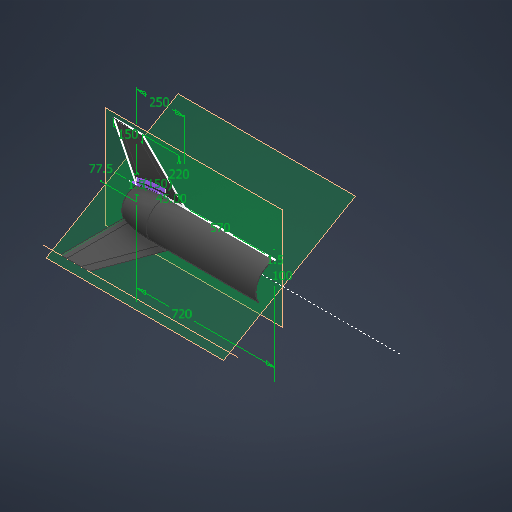
# Autodesk Inventor part: 26P0131-04-0005-AY
Saved by Autodesk Inventor 2026.1 (Build 301233020, 233B)
## iProperties
Created: 2026-01-29
Part Number: 26P0131-04-0005-AY
Material: CFRP
Document SubType Name: Modeling
Designer: User
Density: 1.43 g/cm^3
Appearance: Carbon Fiber
Author: User
Autodesk Inventor part; units mm, degrees
ref_plane "YZ Plane" through (0, 0, 0) normal (1, 0, 0) x (0, 1, 0)
ref_plane "XZ Plane" through (0, 0, 0) normal (0, 1, 0) x (-1, 0, 0)
ref_plane "XY Plane" through (0, 0, 0) normal (0, 0, 1) x (1, 0, 0)
sketch "Sketch3" plane through (0, 0, 0) normal (0, 0, 1) x (1, 0, 0)
  spline S0 degree 4 poles (0, 76) (3.2261, 76.9678) (7.7454, 78.2848) (13.5618, 79.9096) (20.6802, 81.7875) (25.8529, 83.0987) (31.0257, 84.3563) (36.1985, 85.5604) (41.3712, 86.7109) (46.544, 87.808) (51.7168, 88.8516) (56.8895, 89.8416) (62.0623, 90.7781) (67.2351, 91.6611) (72.4079, 92.4906) (77.5807, 93.2666) (82.7535, 93.9891) (87.9263, 94.658) (93.0991, 95.2734) (98.2719, 95.8353) (103.4447, 96.3438) (108.6175, 96.7986) (113.7903, 97.2) (118.9631, 97.5479) (124.1359, 97.8422) (129.3087, 98.083) (136.4207, 98.3405) (142.2404, 98.461) (146.767, 98.5) (150, 98.5) knots 0 0 0 0 0 0.087261 0.122096 0.156887 0.191635 0.226341 0.261008 0.295637 0.33023 0.364788 0.399313 0.433807 0.468271 0.502708 0.537118 0.571504 0.605867 0.64021 0.674533 0.708839 0.74313 0.777407 0.811672 0.845927 0.880174 0.914415 1 1 1 1 1
  spline S1 degree 4 poles (0, 77.5) (3.2261, 78.4678) (7.7454, 79.7848) (13.5618, 81.4096) (20.6802, 83.2875) (25.8529, 84.5987) (31.0257, 85.8563) (36.1985, 87.0604) (41.3712, 88.2109) (46.544, 89.308) (51.7168, 90.3516) (56.8895, 91.3416) (62.0623, 92.2781) (67.2351, 93.1611) (72.4079, 93.9906) (77.5807, 94.7666) (82.7535, 95.4891) (87.9263, 96.158) (93.0991, 96.7734) (98.2719, 97.3353) (103.4447, 97.8438) (108.6175, 98.2986) (113.7903, 98.7) (118.9631, 99.0479) (124.1359, 99.3422) (129.3087, 99.583) (136.4207, 99.8405) (142.2404, 99.961) (146.767, 100) (150, 100) knots 0 0 0 0 0 0.087261 0.122096 0.156887 0.191635 0.226341 0.261008 0.295637 0.33023 0.364788 0.399313 0.433807 0.468271 0.502708 0.537118 0.571504 0.605867 0.64021 0.674533 0.708839 0.74313 0.777407 0.811672 0.845927 0.880174 0.914415 1 1 1 1 1
  line L0 (0, 77.5) -> (0, 76)
  line L1 (150, 100) -> (720, 100)
  line L2 (150, 98.5) -> (720, 98.5)
  line L3 (720, 100) -> (720, 98.5)
  line L4 (0, 0) -> (1383.1618, 0) construction
  line L5 (250, 100) -> (30, 320)
  line L6 (30, 320) -> (-120, 320)
  line L7 (-120, 320) -> (0, 77.5)
  point P0 (5.1724, 77.525)
  point P1 (10.3448, 78.9964)
  point P2 (15.5172, 80.4144)
  point P3 (20.6897, 81.7788)
  point P4 (25.8621, 83.0898)
  point P5 (31.0345, 84.3472)
  point P6 (36.2069, 85.5511)
  point P7 (41.3793, 86.7015)
  point P8 (46.5517, 87.7985)
  point P9 (51.7241, 88.8419)
  point P10 (56.8966, 89.8317)
  point P11 (62.069, 90.7681)
  point P12 (67.2414, 91.651)
  point P13 (72.4138, 92.4804)
  point P14 (77.5862, 93.2562)
  point P15 (82.7586, 93.9786)
  point P16 (87.931, 94.6474)
  point P17 (93.1034, 95.2628)
  point P18 (98.2759, 95.8246)
  point P19 (103.4483, 96.3329)
  point P20 (108.6207, 96.7878)
  point P21 (113.7931, 97.1891)
  point P22 (118.9655, 97.5369)
  point P23 (124.1379, 97.8312)
  point P24 (129.3103, 98.0719)
  point P25 (134.4828, 98.2592)
  point P26 (139.6552, 98.393)
  point P27 (144.8276, 98.4732)
  point P28 (5.1724, 79.025)
  point P29 (10.3448, 80.4964)
  point P30 (15.5172, 81.9144)
  point P31 (20.6897, 83.2788)
  point P32 (25.8621, 84.5898)
  point P33 (31.0345, 85.8472)
  point P34 (36.2069, 87.0511)
  point P35 (41.3793, 88.2015)
  point P36 (46.5517, 89.2985)
  point P37 (51.7241, 90.3419)
  point P38 (56.8966, 91.3317)
  point P39 (62.069, 92.2681)
  point P40 (67.2414, 93.151)
  point P41 (72.4138, 93.9804)
  point P42 (77.5862, 94.7562)
  point P43 (82.7586, 95.4786)
  point P44 (87.931, 96.1474)
  point P45 (93.1034, 96.7628)
  point P46 (98.2759, 97.3246)
  point P47 (103.4483, 97.8329)
  point P48 (108.6207, 98.2878)
  point P49 (113.7931, 98.6891)
  point P50 (118.9655, 99.0369)
  point P51 (124.1379, 99.3312)
  point P52 (129.3103, 99.5719)
  point P53 (134.4828, 99.7592)
  point P54 (139.6552, 99.893)
  point P55 (144.8276, 99.9732)
  dimension "d6" = 570
  dimension "d7" = 1.5
  dimension "d8" = 1.5
  dimension "d9" = 100
  dimension "d11" = 45
  dimension "d12" = 220
  dimension "d13" = 250
  dimension "d14" = 150
  dimension "d15" = 77.5
  dimension "d63" = 720
  dimension "d66" = 150
  constraints: 16 end point, 4 horizontal, 2 vertical, 1 parallel, 1 point on line, 1 vertical alignment, 60 other
  measures "d6" distance of L1.start L1.end
  measures "d7" distance of L1.end L2.end
  measures "d8" distance of L0.start L0.end
  measures "d9" distance from line of L4 L1.end
  measures "d11" angle of L1 L5
  measures "d12" horizontal distance of L5.start L5.end
  measures "d13" horizontal distance of L5.start L4.start
  measures "d14" distance of L5.end L6.end
  measures "d15" distance of L4.start L0.start
  measures "d63" horizontal distance of L4.start L2.end
  measures "d66" horizontal distance of L2.start L4.start
revolve "Revolution1" add sketch "Sketch3" angle 360 about axis through (0, 0, 0) along (1, 0, 0) contours L0 S1 L1 L3 L2 S0
extrude "Extrusion1" add sketch "Sketch3" along normal mid plane 3 contours L7 L6 L5 L1 S1
pattern_circular "Circular Pattern1" count 3 over 360 about axis through (-10, 0, 0) along (-1, 0, 0) of "Extrusion1"
chamfer "Chamfer1" distance 30 distance2 1.5 1 edges at (140, -103.701, 182.6153) measured on face at (-30, -118.2843, 207.8744)
chamfer "Chamfer2" distance 30 distance2 1.5 1 edges at (140, -106.299, 181.1153) measured on face at (-30, -120.8824, 206.3744)
chamfer "Chamfer3" distance 30 distance2 1.5 1 edges at (-60, -98.076, 172.8725) measured on face at (-44.1421, -118.2843, 207.8744)
chamfer "Chamfer5" distance 30 distance2 1.5 1 edges at (-60, 198.75, 1.5) measured on face at (-30, 239.1667, 1.5)
chamfer "Chamfer6" distance 30 distance2 1.5 1 edges at (140, 210, 1.5) measured on face at (-9.0023, 241.8283, 1.5)
chamfer "Chamfer7" distance 30 distance2 1.5 1 edges at (-60, 198.75, -1.5) measured on face at (-30, 239.1667, -1.5)
chamfer "Chamfer8" distance 30 distance2 1.5 1 edges at (140, 210, -1.5) measured on face at (-9.0027, 241.8282, -1.5)
chamfer "Chamfer9" distance 30 distance2 1.5 1 edges at (-60, -98.076, -172.8725) measured on face at (-30, -118.2843, -207.8744)
chamfer "Chamfer10" distance 30 distance2 1.5 1 edges at (140, -103.701, -182.6153) measured on face at (-9.0023, -119.6151, -210.1794)
chamfer "Chamfer11" distance 30 distance2 1.5 1 edges at (140, -106.299, -181.1153) measured on face at (-30, -120.8824, -206.3744)
chamfer "Chamfer12" distance 30 distance2 1.5 1 edges at (-60, -100.674, -171.3725) measured on face at (-44.1419, -120.8824, -206.3744)
chamfer "Chamfer13" distance 30 distance2 1.5 1 edges at (-60, -100.674, 171.3725) measured on face at (-44.1419, -120.8824, 206.3744)
ref_plane "Work Plane1" through (30, 320, 0) normal (0, 0, -1) x (-1, 0, 0)
ref_plane "Work Plane2" through (-120, -160, 277.1281) normal (0, -0.866, -0.5) x (1, 0, 0)
split "Split1" plane through (-120, -160, 277.1281) removes the side toward (0, -0.866, -0.5)
split "Split2" plane through (30, 320, 0) removes the side toward (0, 0, -1)
body "Solid1"
